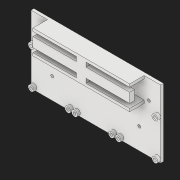
# Autodesk Inventor part: BP003
Saved by Autodesk Inventor 2017 SP1 (Build 210196100, 196)
## iProperties
Created: 2018-01-03
Part Number: BP003
Material: ABS Plastic
Document SubType Name: Modeling
Designer: Zach
Density: 1.06 g/cm^3
Appearance: CR White
Author: Zach
Autodesk Inventor part; units mm, degrees
ref_plane "YZ Plane" through (0, 0, 0) normal (1, 0, 0) x (0, 1, 0)
ref_plane "XZ Plane" through (0, 0, 0) normal (0, 1, 0) x (-1, 0, 0)
ref_plane "XY Plane" through (0, 0, 0) normal (0, 0, 1) x (1, 0, 0)
sketch "Sketch1" plane through (0, 0, 0) normal (0, 0, 1) x (1, 0, 0)
  line L0 (0, 44) -> (44, 44) construction
  line L1 (44, 44) -> (44, 0) construction
  line L2 (44, 0) -> (0, 0) construction
  line L3 (0, 0) -> (0, 44) construction
  line L4 (3, 41) -> (41, 41) construction
  line L5 (41, 41) -> (41, 3) construction
  line L6 (41, 3) -> (3, 3) construction
  line L7 (3, 3) -> (3, 41) construction
  circle A0 centre (3, 41) radius 1.5
  circle A1 centre (41, 41) radius 1.5
  circle A2 centre (41, 3) radius 1.5
  circle A3 centre (3, 3) radius 1.5
  line L8 (44, 3) -> (44, 44) construction
  line L9 (48, 41) -> (86, 41) construction
  line L10 (86, 41) -> (86, 3) construction
  line L11 (86, 3) -> (48, 3) construction
  line L12 (48, 3) -> (48, 41) construction
  circle A4 centre (48, 41) radius 1.5
  circle A5 centre (48, 3) radius 1.5
  circle A6 centre (86, 3) radius 1.5
  circle A7 centre (86, 41) radius 1.5
  line L13 (45, 44) -> (89, 44) construction
  line L14 (89, 44) -> (89, 0) construction
  line L15 (89, 0) -> (45, 0) construction
  line L16 (45, 0) -> (45, 44) construction
  line L17 (90, 44) -> (134, 44) construction
  line L18 (134, 44) -> (134, 0) construction
  line L19 (134, 0) -> (90, 0) construction
  line L20 (90, 0) -> (90, 44) construction
  line L21 (93, 41) -> (131, 41) construction
  line L22 (131, 41) -> (131, 3) construction
  line L23 (131, 3) -> (93, 3) construction
  line L24 (93, 3) -> (93, 41) construction
  circle A8 centre (93, 41) radius 1.5
  circle A9 centre (131, 41) radius 1.5
  circle A10 centre (131, 3) radius 1.5
  circle A11 centre (93, 3) radius 1.5
  line L25 (0, 0) -> (134, 0)
  line L26 (134, 0) -> (134, 44)
  line L27 (0, 44) -> (0, 0)
  line L28 (0, 44) -> (134, 44)
  point P0 (0, 0)
  point P1 (22, 41)
  point P2 (41, 22)
  point P3 (44, 22)
  point P4 (22, 44)
  point P5 (67, 41)
  point P6 (67, 44)
  point P7 (86, 22)
  point P8 (89, 22)
  point P9 (112, 41)
  point P10 (112, 44)
  point P11 (131, 22)
  point P12 (134, 22)
  dimension "d9" = 44
  dimension "d10" = 44
  dimension "d11" = 38
  dimension "d12" = 38
  dimension "d17" = 3
  dimension "d18" = 3
  dimension "d19" = 3
  dimension "d20" = 3
  dimension "d33" = 38
  dimension "d34" = 38
  dimension "d35" = 3
  dimension "d36" = 3
  dimension "d37" = 3
  dimension "d38" = 3
  dimension "d39" = 44
  dimension "d40" = 44
  dimension "d41" = 1
  dimension "d42" = 44
  dimension "d43" = 44
  dimension "d44" = 38
  dimension "d45" = 38
  dimension "d46" = 1
  dimension "d47" = 3
  dimension "d48" = 3
  dimension "d49" = 3
  dimension "d50" = 3
  constraints: 58 end point, 13 coincident, 13 parallel, 12 centre point, 12 midpoint, 7 horizontal, 6 perpendicular, 5 horizontal alignment, 3 vertical alignment, 1 collinear
  measures "d9" distance of L1.end L2.end
  measures "d10" distance of L0.end L1.end
  measures "d11" distance of L5.end L6.end
  measures "d12" distance of L4.end L5.end
  measures "d17" diameter of A0
  measures "d18" diameter of A1
  measures "d19" diameter of A2
  measures "d20" diameter of A3
  measures "d33" distance of L10.end L11.end
  measures "d34" distance of L9.end L10.end
  measures "d35" diameter of A4
  measures "d36" diameter of A5
  measures "d37" diameter of A6
  measures "d38" diameter of A7
  measures "d39" distance of L14.end L15.end
  measures "d40" distance of L13.end L14.end
  measures "d41" distance between parallel lines of L8 L16
  measures "d42" distance of L18.end L19.end
  measures "d43" distance of L17.end L18.end
  measures "d44" distance of L22.end L23.end
  measures "d45" distance of L21.end L22.end
  measures "d46" distance between parallel lines of L14 L20
  measures "d47" diameter of A8
  measures "d48" diameter of A9
  measures "d49" diameter of A10
  measures "d50" diameter of A11
extrude "Extrusion1" add sketch "Sketch1" along normal blind 3
sketch "Sketch2" plane through (0, 0, 3) normal (0, 0, 1) x (1, 0, 0)
  circle A0 centre (93, 3) radius 1.5 projected
  circle A1 centre (131, 3) radius 1.5 projected
  circle A2 centre (131, 41) radius 1.5 projected
  circle A3 centre (93, 41) radius 1.5 projected
  circle A4 centre (86, 41) radius 1.5 projected
  circle A5 centre (86, 3) radius 1.5 projected
  circle A6 centre (48, 3) radius 1.5 projected
  circle A7 centre (48, 41) radius 1.5 projected
  circle A8 centre (3, 3) radius 1.5 projected
  circle A9 centre (41, 3) radius 1.5 projected
  circle A10 centre (41, 41) radius 1.5 projected
  circle A11 centre (3, 41) radius 1.5 projected
  line L0 (0, 44) -> (0, 0) construction
  line L1 (0, 0) -> (134, 0) construction
  line L2 (134, 0) -> (134, 44) construction
  circle A12 centre (131, 41) radius 1.5 projected
  circle A13 centre (131, 41) radius 3
  circle A14 centre (131, 3) radius 3
  circle A15 centre (93, 3) radius 3
  circle A16 centre (86, 3) radius 3
  circle A17 centre (48, 3) radius 3
  circle A18 centre (41, 3) radius 1.5 projected
  circle A19 centre (41, 3) radius 3
  circle A20 centre (3, 3) radius 1.5 projected
  circle A21 centre (3, 3) radius 3
  circle A22 centre (3, 41) radius 1.5 projected
  circle A23 centre (3, 41) radius 3
  circle A24 centre (41, 41) radius 1.5 projected
  circle A25 centre (41, 41) radius 3
  circle A26 centre (48, 41) radius 1.5 projected
  circle A27 centre (48, 41) radius 3
  circle A28 centre (93, 41) radius 3
  circle A29 centre (86, 41) radius 3
  line L3 (134, 44) -> (0, 44) projected
  point P0 (0, 0)
  dimension "d70" = 6
  dimension "d71" = 6
  dimension "d72" = 6
  dimension "d73" = 6
  dimension "d74" = 6
  dimension "d75" = 6
  dimension "d76" = 6
  dimension "d77" = 6
  dimension "d79" = 6
  dimension "d80" = 6
  dimension "d83" = 6
  dimension "d84" = 6
  constraints: 12 centre point, 12 coincident
  measures "d70" diameter of A13
  measures "d71" diameter of A14
  measures "d72" diameter of A15
  measures "d73" diameter of A16
  measures "d74" diameter of A17
  measures "d75" diameter of A19
  measures "d76" diameter of A21
  measures "d77" diameter of A23
  measures "d79" diameter of A25
  measures "d80" diameter of A27
  measures "d83" diameter of A28
  measures "d84" diameter of A29
extrude "Extrusion2" add sketch "Sketch2" along normal blind 3
sketch "Sketch3" plane through (0, 0, 0) normal (0, 0, -1) x (-1, 0, 0)
  line L0 (0, 44) -> (0, 0) projected
  line L1 (0, 44) -> (-134, 44)
  line L2 (-134, 44) -> (-134, 70)
  line L3 (-134, 70) -> (0, 70)
  line L4 (0, 70) -> (0, 44)
  dimension "d87" = 26
  constraints: 8 end point, 2 parallel, 1 coincident, 1 horizontal, 1 perpendicular
  measures "d87" distance of L1.end L2.end
extrude "Extrusion3" add sketch "Sketch3" against normal blind 3
sketch "Sketch4" plane through (0, 0, 3) normal (0, 0, 1) x (1, 0, 0)
  line L0 (0, 70) -> (0, 0) projected
  line L1 (134, 0) -> (134, 70) projected
  line L2 (0, 70) -> (134, 70)
  line L3 (134, 70) -> (134, 67)
  line L4 (134, 67) -> (0, 67)
  line L5 (0, 67) -> (0, 70)
  line L6 (0, 45) -> (134, 45)
  line L7 (134, 45) -> (134, 48)
  line L8 (134, 48) -> (0, 48)
  line L9 (0, 48) -> (0, 45)
  line L10 (93, 0) -> (131, 0) projected
  line L11 (62, 48) -> (72, 48)
  line L12 (72, 48) -> (72, 67)
  line L13 (72, 67) -> (62, 67)
  line L14 (62, 67) -> (62, 48)
  point P0 (67, 67)
  dimension "d90" = 3
  dimension "d91" = 3
  dimension "d92" = 45
  dimension "d101" = 10
  constraints: 24 end point, 6 parallel, 5 point on line, 3 horizontal, 3 perpendicular, 2 midpoint
  measures "d90" distance of L2.end L3.end
  measures "d91" distance of L7.end L6.end
  measures "d92" distance between parallel lines of L10 L6
  measures "d101" distance between parallel lines of L12 L14
extrude "Extrusion4" add sketch "Sketch4" along normal blind 15 contours L2 L1 L4 L0 | L8 L1 L6 L0 | L4 L12 L8 L14
sketch "Sketch5" plane through (0, 0, 18) normal (0, 0, 1) x (1, 0, 0)
  line L0 (62, 67) -> (62, 48) projected
  line L1 (62, 62.5) -> (0, 62.5)
  line L2 (0, 62.5) -> (0, 52.5)
  line L3 (0, 52.5) -> (62, 52.5)
  line L4 (62, 52.5) -> (62, 62.5)
  line L5 (0, 67) -> (0, 48) projected
  line L6 (72, 48) -> (72, 67) projected
  line L7 (134, 0) -> (134, 70) projected
  line L8 (72, 62.5) -> (134, 62.5)
  line L9 (134, 62.5) -> (134, 52.5)
  line L10 (134, 52.5) -> (72, 52.5)
  line L11 (72, 52.5) -> (72, 62.5)
  point P0 (0, 0)
  point P1 (0, 57.5)
  point P2 (62, 57.5)
  point P3 (72, 57.5)
  dimension "d97" = 10
  dimension "d98" = 10
  constraints: 16 end point, 6 midpoint, 4 parallel, 3 point on line, 2 horizontal, 2 perpendicular
  measures "d97" distance of L2.end L1.end
  measures "d98" distance between parallel lines of L10 L8
extrude "Extrusion5" add sketch "Sketch5" against normal blind 5
sketch "Sketch6" plane through (0, 0, 18) normal (0, 0, 1) x (1, 0, 0)
  line L0 (72, 67) -> (134, 67) projected
  line L1 (72, 48) -> (134, 48) projected
  line L2 (72, 67) -> (117, 67)
  line L3 (117, 67) -> (117, 48)
  line L4 (117, 48) -> (72, 48)
  line L5 (72, 48) -> (72, 67)
  line L6 (134, 0) -> (134, 70) projected
  line L7 (134, 70) -> (117, 70)
  line L8 (117, 70) -> (117, 45)
  line L9 (117, 45) -> (134, 45)
  line L10 (134, 45) -> (134, 70)
  line L11 (0, 45) -> (134, 45) projected
  line L12 (0, 48) -> (62, 48) projected
  line L13 (62, 67) -> (17, 67)
  line L14 (17, 67) -> (17, 48)
  line L15 (17, 48) -> (62, 48)
  line L16 (62, 48) -> (62, 67)
  line L17 (0, 70) -> (0, 67) projected
  line L18 (0, 70) -> (17, 70)
  line L19 (17, 70) -> (17, 45)
  line L20 (17, 45) -> (0, 45)
  line L21 (0, 45) -> (0, 70)
  point P0 (0, 0)
  dimension "d102" = 45
  dimension "d103" = 45
  constraints: 32 end point, 8 parallel, 6 point on line, 4 horizontal, 4 perpendicular, 1 coincident
  measures "d102" distance of L3.end L4.end
  measures "d103" distance of L15.end L14.end
extrude "Extrusion6" cut sketch "Sketch6" against normal through all contours L8 L7 L6 L0 | L0 L6 L1 L3 | L1 L6 L9 L8 | L21 L12 L19 L11 | L21 L17 L18 L19 L14 L12
sketch "Sketch7" plane through (0, 0, 3) normal (0, 0, 1) x (1, 0, 0)
  circle A0 centre (12, 50) radius 1.5
  circle A1 centre (122, 50) radius 1.5
  line L0 (17, 67) -> (17, 48) projected
  line L1 (17, 45) -> (0, 45) projected
  line L2 (117, 48) -> (117, 67) projected
  line L3 (17, 48) -> (17, 45) projected
  line L4 (17, 45) -> (7, 45)
  line L5 (7, 45) -> (7, 55)
  line L6 (7, 55) -> (17, 55)
  line L7 (17, 55) -> (17, 45)
  line L8 (117, 45) -> (17, 45) projected
  line L9 (117, 45) -> (127, 45)
  line L10 (127, 45) -> (127, 55)
  line L11 (127, 55) -> (117, 55)
  line L12 (117, 55) -> (117, 45)
  point P0 (0, 0)
  dimension "d106" = 3
  dimension "d107" = 3
  dimension "d108" = 5
  dimension "d109" = 5
  dimension "d110" = 5
  dimension "d111" = 10
  dimension "d112" = 10
  dimension "d113" = 10
  dimension "d114" = 10
  constraints: 16 end point, 4 parallel, 2 centre point, 2 horizontal, 2 perpendicular, 1 horizontal alignment
  measures "d106" diameter of A0
  measures "d107" diameter of A1
  measures "d108" distance from line of L0 A0.centre
  measures "d109" distance from line of L1 A0.centre
  measures "d110" distance from line of L2 A1.centre
  measures "d111" distance of L5.end L6.end
  measures "d112" distance of L4.end L5.end
  measures "d113" distance of L11.end L10.end
  measures "d114" distance of L10.end L9.end
extrude "Extrusion7" add sketch "Sketch7" against normal blind 3
sketch "Sketch8" plane through (0, 0, 3) normal (0, 0, 1) x (1, 0, 0)
  circle A0 centre (22, 22) radius 1.5
  circle A1 centre (112, 22) radius 1.5
  circle A2 centre (3, 41) radius 1.5 construction
  line L0 (3, 41) -> (3, 3) construction
  line L1 (3, 41) -> (41, 41) construction
  circle A3 centre (93, 41) radius 1.5 construction
  line L2 (93, 41) -> (131, 41) construction
  circle A4 centre (41, 41) radius 1.5 construction
  circle A5 centre (131, 41) radius 1.5 construction
  circle A6 centre (3, 3) radius 1.5 construction
  point P0 (0, 0)
  point P1 (3, 22)
  point P2 (112, 41)
  point P3 (22, 41)
  dimension "d117" = 3
  dimension "d118" = 3
  constraints: 6 end point, 3 coincident, 3 midpoint, 2 centre point, 2 horizontal, 2 horizontal alignment, 2 vertical alignment, 1 vertical
  measures "d117" diameter of A0
  measures "d118" diameter of A1
extrude "Extrusion8" cut sketch "Sketch8" against normal through all
sketch "Sketch9" plane through (0, 0, 0) normal (0, 0, -1) x (-1, 0, 0)
  line L0 (-134, 41) -> (-134, 45) projected
  line L1 (-134, 45) -> (-134, 70)
  line L2 (-117, 70) -> (-17, 70) projected
  line L3 (-117, 70) -> (-134, 70)
  line L4 (-127, 55) -> (-127, 45) projected
  line L5 (-127, 45) -> (-134, 45) projected
  line L6 (-117, 70) -> (-117, 55) projected
  line L7 (-117, 55) -> (-127, 55) projected
  line L8 (-17, 55) -> (-17, 70) projected
  line L9 (-7, 55) -> (-17, 55) projected
  line L10 (-7, 45) -> (-7, 55) projected
  line L11 (0, 45) -> (-7, 45) projected
  line L12 (0, 45) -> (0, 0) projected
  line L13 (0, 45) -> (0, 70)
  line L14 (0, 70) -> (-17, 70)
  constraints: 8 end point, 2 vertical, 1 collinear, 1 perpendicular
extrude "Extrusion9" add sketch "Sketch9" against normal blind 3
body "Solid1"
